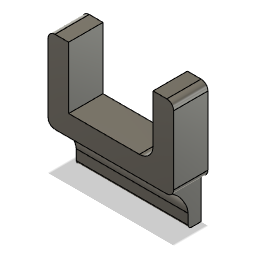
holder v3 (Autodesk Fusion 360 design; units mm, degrees)
Autodesk Fusion 360 part; units mm, degrees
sketch "Sketch1" plane through (0, 0, 0) normal (0, 1, 0) x (1, 0, 0)
  line L0 (0, 0) -> (18.3, 0)
  line L1 (18.3, 0) -> (18.3, -5)
  line L2 (18.3, -5) -> (0, -5)
  line L3 (0, -5) -> (0, 0)
  dimension "d1" = 18.3
  dimension "d2" = 5
  constraint horizontal L0
  constraint vertical L1
  constraint horizontal L2
  constraint vertical L3
  constraint coincident L0.start L3.end
  measures "d1" distance of L0.start L0.end
  measures "d2" distance of L0.start L2.end
extrude "Extrude1" add sketch "Sketch1" along normal blind 3
sketch "Sketch2" plane through (0, 3, 0) normal (0, 1, 0) x (-1, 0, 0)
  line L0 (0, 5) -> (-18.3, 5)
  line L1 (-18.3, 5) -> (-18.3, 0)
  line L2 (-18.3, 0) -> (0, 0)
  line L3 (0, 0) -> (0, 5)
  line L4 (0, 0) -> (-3, 0)
  line L5 (-3, 0) -> (-3, 5)
  line L6 (-3, 5) -> (0, 5)
  line L7 (0, 5) -> (0, 0)
  line L8 (-18.3, 0) -> (-15.3, 0)
  line L9 (-15.3, 0) -> (-15.3, 5)
  line L10 (-15.3, 5) -> (-18.3, 5)
  line L11 (-18.3, 5) -> (-18.3, 0)
  dimension "d5" = 3
  dimension "d6" = 3
  dimension "d7" = 5
  constraint horizontal L4
  constraint vertical L5
  constraint horizontal L6
  constraint vertical L7
  constraint coincident L2.end L3.start
  constraint horizontal L8
  constraint vertical L9
  constraint horizontal L10
  constraint vertical L11
  constraint coincident L1.end L2.start
  measures "d5" distance of L2.end L4.end
  measures "d6" distance of L1.end L8.end
  measures "d7" distance of L1.end L0.end
extrude "Extrude2" add sketch "Sketch2" along normal blind 9 contours L0 L2 L3 L4 L5 L6 L7 | L0 L1 L2 L8 L9 L10 L11
fillet "Fillet1" radius 2 1 edges at (15.3, 3, 2.5)
fillet "Fillet2" radius 1 4 edges at (0, 0, 2.5) (18.3, 0, 2.5) (0, 12, 2.5) (18.3, 12, 2.5)
extrude "Extrude3" add 1 faces at (6.4333, 0, 1.6667) along direction (0, -1, 0) blind 4
sketch "Sketch3" plane through (17.3, 0, 0) normal (1, 0, 0) x (0, 0, -1)
  line L0 (0, 0) -> (-5, 0)
  line L1 (-5, 0) -> (-5, -4)
  line L2 (-5, -4) -> (0, -4)
  line L3 (0, -4) -> (0, 0)
  line L4 (-2.5, 0) -> (-2.5, -4) construction
  spline S0 degree 5 poles (-5, 0) (-4.9471, -0.0246) (-4.844, -0.0733) (-4.6979, -0.1449) (-4.5202, -0.2376) (-4.3258, -0.349) (-4.157, -0.4565) (-4.0094, -0.5614) (-3.8742, -0.666) (-3.7405, -0.7738) (-3.6051, -0.8883) (-3.4674, -1.0128) (-3.3291, -1.1499) (-3.192, -1.3006) (-3.0571, -1.4644) (-2.9245, -1.6395) (-2.7947, -1.8235) (-2.6678, -2.0138) (-2.5446, -2.208) (-2.4267, -2.4046) (-2.316, -2.6025) (-2.2148, -2.8012) (-2.1251, -3.0004) (-2.0487, -3.1999) (-1.9864, -3.3996) (-1.9389, -3.5995) (-1.9129, -3.7596) (-1.9, -3.8798) (-1.8945, -3.9599) (-1.8924, -4) knots 0 0 0 0 0 0 0.04 0.08 0.12 0.16 0.2 0.24 0.28 0.32 0.36 0.4 0.44 0.48 0.52 0.56 0.6 0.64 0.68 0.72 0.76 0.8 0.84 0.88 0.92 0.96 1 1 1 1 1 1
  line L5 (-4.3837, -0.2829) -> (-3.5871, -0.8801)
  point P0 (-3.9854, -0.5815)
  point P1 (-3.3558, -1.126)
  point P2 (-2.6836, -1.992)
  point P3 (-2.1229, -3.0139)
  constraint midpoint L0 L4.start
  constraint midpoint L2 L4.end
  constraint coincident L0.end L1.start
  constraint coincident L2 S0.end
  constraint midpoint P0 L5
extrude "Extrude4" cut sketch "Sketch3" against normal blind 68 contours L1 L2 S0
extrude "Extrude5" add 1 faces at (6.4333, -4, 0.6308) along direction (0, -1, 0) blind 2
fillet "Fillet3" radius 0.5 1 edges at (9.15, -6, 1.8924)
equation "d1 = 12.3 mm + 6 mm"
